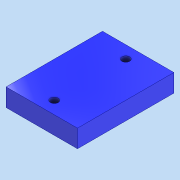
# Autodesk Inventor part: ir_sensor_cap
Saved by Autodesk Inventor 2022 (Build 260153000, 153)
## iProperties
Created: 2021-09-16
Part Number: ir_sensor_cap
Material: Generic
Document SubType Name: Modeling
Designer: nnico
Density: 1 g/cm^3
Appearance: Blue - Wall Paint - Glossy
Author: nnico
Autodesk Inventor part; units mm, degrees
ref_plane "YZ Plane" through (0, 0, 0) normal (1, 0, 0) x (0, 1, 0)
ref_plane "XZ Plane" through (0, 0, 0) normal (0, 1, 0) x (-1, 0, 0)
ref_plane "XY Plane" through (0, 0, 0) normal (0, 0, 1) x (1, 0, 0)
sketch "Sketch5" plane through (0, 0, 0) normal (0, 1, 0) x (-1, 0, 0)
  line L0 (10, 13.5) -> (-10, 13.5)
  line L1 (-10, 13.5) -> (-10, -13.5)
  line L2 (-10, -13.5) -> (10, -13.5)
  line L3 (10, -13.5) -> (10, 13.5)
  line L4 (0, 13.5) -> (0, -13.5) construction
  line L5 (10, 0) -> (-10, 0) construction
  circle A0 centre (0, 10) radius 1.1
  circle A1 centre (0, -10) radius 1.1
  point P0 (0, 0)
  point P1 (0, 0)
  point P2 (0, 0)
  dimension "d12" = 20
  dimension "d13" = 27
  dimension "d14" = 2.2
  dimension "d15" = 3.5
  constraints: 12 end point, 5 midpoint, 2 centre point, 2 coincident, 2 parallel, 1 horizontal, 1 perpendicular, 1 point on line, 1 symmetric about line, 1 other
  measures "d12" distance of L2.end L1.end
  measures "d13" distance of L1.end L0.end
  measures "d14" diameter of A0
  measures "d15" distance from line of L0 A0.centre
extrude "Extrusion4" add sketch "Sketch5" along normal blind 5
body "Solid2"
